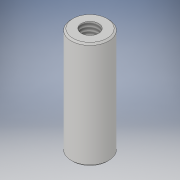
# Autodesk Inventor part: Distanzhülse_M4x20
Saved by Autodesk Inventor 2018 (Build 220112000, 112)
## iProperties
Created: 2017-12-09
Part Number: Distanzhülse_M4x20
Material: Generisch
Document SubType Name: Modeling
Designer: aXe
Density: 1 g/cm^3
Appearance: Vorgabe
Author: aXe
Länge: 20,000 mm
Durchmesser: 7,000 mm
Autodesk Inventor part; units mm, degrees
ref_plane "YZ Plane" through (0, 0, 0) normal (1, 0, 0) x (0, 1, 0)
ref_plane "XZ Plane" through (0, 0, 0) normal (0, 1, 0) x (-1, 0, 0)
ref_plane "XY Plane" through (0, 0, 0) normal (0, 0, 1) x (1, 0, 0)
sketch "Skizze1" plane through (0, 0, 0) normal (0, 0, 1) x (1, 0, 0)
  circle A0 centre (0, 0) radius 3.5
  dimension "d0" = 7
  constraints: 1 centre point, 1 coincident
  measures "d0" diameter of A0
extrude "Extrusion1" add sketch "Skizze1" along normal mid plane 20
chamfer "Fase1" distance 0.3 angle 45 2 edges at (-3.5, 0, 10) (-3.5, 0, -10)
hole "Bohrung1" at (0, 0, 10) direction (0, 0, -1) diameter 3.242 end through all thread size "M4x0.7" class "6H" standard "ANSI Metric M Profile"
equation "\"d0\" = Durchmesser"
equation "\"d1\" = Länge"
equation "\"d9\" = Länge"
equation "\"Länge\" = 20"
equation "\"Durchmesser\" = 7"
